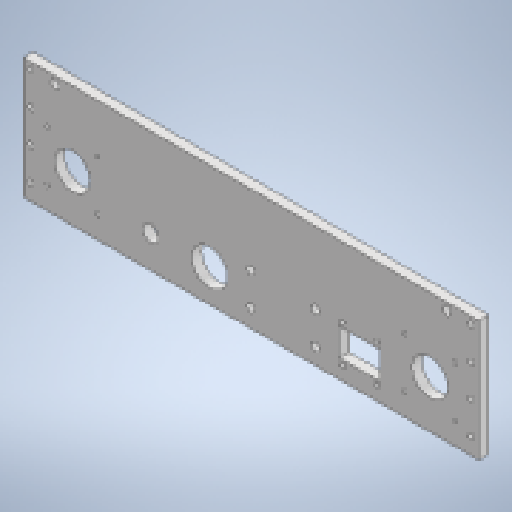
# Autodesk Inventor part: креп_мотора
Saved by Autodesk Inventor 2023.1 (Build 271208000, 208)
## iProperties
Created: 2025-12-22
Part Number: креп_мотора
Material: Типовые
Document SubType Name: Modeling
Designer: DELL
Density: 1 g/cm^3
Appearance: По умолчанию
Author: DELL
Autodesk Inventor part; units mm, degrees
ref_plane "YZ Plane" through (0, 0, 0) normal (1, 0, 0) x (0, 1, 0)
ref_plane "XZ Plane" through (0, 0, 0) normal (0, 1, 0) x (-1, 0, 0)
ref_plane "XY Plane" through (0, 0, 0) normal (0, 0, 1) x (1, 0, 0)
sketch "Эскиз1" plane through (0, 0, 0) normal (0, 0, 1) x (1, 0, 0)
  line L0 (-26.0621, -17.2379) -> (-22.2379, -21.0621) projected
  arc A0 (-22.2379, -21.0621) -> (-22.0257, -21.15) centre (-22.0257, -20.85) ccw projected
  line L1 (-22.0257, -21.15) -> (12.0257, -21.15) projected
  arc A1 (12.0257, -21.15) -> (12.2379, -21.0621) centre (12.0257, -20.85) ccw projected
  line L2 (12.2379, -21.0621) -> (16.0621, -17.2379) projected
  arc A2 (16.0621, -17.2379) -> (16.15, -17.0257) centre (15.85, -17.0257) ccw projected
  line L3 (16.15, -17.0257) -> (16.15, 17.0257) projected
  arc A3 (16.15, 17.0257) -> (16.0621, 17.2379) centre (15.85, 17.0257) ccw projected
  line L4 (16.0621, 17.2379) -> (12.2379, 21.0621) projected
  arc A4 (12.2379, 21.0621) -> (12.0257, 21.15) centre (12.0257, 20.85) ccw projected
  line L5 (12.0257, 21.15) -> (-22.0257, 21.15) projected
  arc A5 (-22.0257, 21.15) -> (-22.2379, 21.0621) centre (-22.0257, 20.85) ccw projected
  line L6 (-22.2379, 21.0621) -> (-26.0621, 17.2379) projected
  arc A6 (-26.0621, 17.2379) -> (-26.15, 17.0257) centre (-25.85, 17.0257) ccw projected
  line L7 (-26.15, 17.0257) -> (-26.15, -17.0257) projected
  arc A7 (-26.15, -17.0257) -> (-26.0621, -17.2379) centre (-25.85, -17.0257) ccw projected
  circle A8 centre (-5, 0) radius 11 projected
  circle A9 centre (-20.5, 15.5) radius 1.25 projected
  circle A10 centre (10.5, 15.5) radius 1.25 projected
  circle A11 centre (10.5, -15.5) radius 1.25 projected
  circle A12 centre (-20.5, -15.5) radius 1.25 projected
  circle A13 centre (20.65, -19.15) radius 1.75 projected
  circle A14 centre (20.65, 0.85) radius 1.75 projected
  circle A15 centre (20.65, 20.85) radius 1.75 projected
  circle A16 centre (20.65, 40.85) radius 1.75 projected
  line L8 (-246.5621, -17.2379) -> (-242.7379, -21.0621) projected
  arc A17 (-242.7379, -21.0621) -> (-242.5257, -21.15) centre (-242.5257, -20.85) ccw projected
  line L9 (-242.5257, -21.15) -> (-208.4743, -21.15) projected
  arc A18 (-208.4743, -21.15) -> (-208.2621, -21.0621) centre (-208.4743, -20.85) ccw projected
  line L10 (-208.2621, -21.0621) -> (-204.4379, -17.2379) projected
  arc A19 (-204.4379, -17.2379) -> (-204.35, -17.0257) centre (-204.65, -17.0257) ccw projected
  line L11 (-204.35, -17.0257) -> (-204.35, 17.0257) projected
  arc A20 (-204.35, 17.0257) -> (-204.4379, 17.2379) centre (-204.65, 17.0257) ccw projected
  line L12 (-204.4379, 17.2379) -> (-208.2621, 21.0621) projected
  arc A21 (-208.2621, 21.0621) -> (-208.4743, 21.15) centre (-208.4743, 20.85) ccw projected
  line L13 (-208.4743, 21.15) -> (-242.5257, 21.15) projected
  arc A22 (-242.5257, 21.15) -> (-242.7379, 21.0621) centre (-242.5257, 20.85) ccw projected
  line L14 (-242.7379, 21.0621) -> (-246.5621, 17.2379) projected
  arc A23 (-246.5621, 17.2379) -> (-246.65, 17.0257) centre (-246.35, 17.0257) ccw projected
  line L15 (-246.65, 17.0257) -> (-246.65, -17.0257) projected
  arc A24 (-246.65, -17.0257) -> (-246.5621, -17.2379) centre (-246.35, -17.0257) ccw projected
  circle A25 centre (-225.5, 0) radius 11 projected
  circle A26 centre (-241, 15.5) radius 1.25 projected
  circle A27 centre (-210, 15.5) radius 1.25 projected
  circle A28 centre (-210, -15.5) radius 1.25 projected
  circle A29 centre (-241, -15.5) radius 1.25 projected
  circle A30 centre (-251.15, -19.15) radius 1.75 projected
  circle A31 centre (-251.15, 0.85) radius 1.75 projected
  circle A32 centre (-251.15, 20.85) radius 1.75 projected
  circle A33 centre (-251.15, 40.85) radius 1.75 projected
  line L16 (-255.45, -29.15) -> (-246.85, -29.15) projected
  line L17 (-255.65, -29.15) -> (-255.65, 270.85) projected
  line L18 (25.15, 270.85) -> (25.15, -29.15) projected
  line L19 (25.15, -29.15) -> (-255.65, -29.15)
  line L20 (-255.65, -29.15) -> (-255.65, 45.35)
  line L21 (-255.65, 45.35) -> (25.15, 45.35)
  line L22 (25.15, 45.35) -> (25.15, -29.15)
  point P0 (25.15, 45.35)
  dimension "d15" = 4.5
  constraints: 8 end point, 2 parallel, 1 horizontal, 1 perpendicular, 1 point on line
  measures "d15" distance from line of L21 A33.centre
extrude "Выдавливание1" add sketch "Эскиз1" along normal blind 6 contours A7 L7 A6 L6 A5 L5 A4 L4 A3 L3 A2 L2 A1 L1 A0 L0 | A24 L15 A23 L14 A22 L13 A21 L12 A20 L11 A19 L10 A18 L9 A17 L8 | L19 L17 L21 L18 L16
sketch "Эскиз2" plane through (0, 0, 6) normal (0, 0, 1) x (1, 0, 0)
  circle A0 centre (20.65, 40.85) radius 1.75 projected
  circle A1 centre (5.65, 40.85) radius 2.6
  circle A2 centre (-236.15, 40.85) radius 2.6
  circle A3 centre (-251.15, 40.85) radius 1.75 projected
  point P0 (0, 0)
  dimension "d16" = 5.2
  dimension "d17" = 15
  dimension "d18" = 5.2
  dimension "d19" = 15
  constraints: 2 centre point
  measures "d16" diameter of A1
  measures "d17" distance of A1.centre A0.centre
  measures "d18" diameter of A2
  measures "d19" distance of A3.centre A2.centre
extrude "Выдавливание2" cut sketch "Эскиз2" against normal blind 6
sketch "Эскиз3" plane through (0, 0, 0) normal (0, 0, -1) x (-1, 0, 0)
  circle A0 centre (115.25, -18.05) radius 2.55
  circle A1 centre (115.25, 1.95) radius 2.55
  line L0 (255.65, 45.35) -> (255.65, -29.15) projected
  point P0 (0, 0)
  dimension "d25" = 5.1
  dimension "d26" = 140.4
  dimension "d27" = 140.4
  constraints: 2 centre point
  measures "d25" diameter of A0
  measures "d26" distance from line of L0 A0.centre
  measures "d27" distance from line of L0 A1.centre
extrude "Выдавливание3" cut sketch "Эскиз3" against normal blind 10
sketch "Эскиз4" plane through (0, 0, 6) normal (0, 0, 1) x (1, 0, 0)
  circle A0 centre (-177.15, -2.65) radius 5 construction
  line L0 (-177.15, -2.65) -> (-177.15, -29.15) construction
  line L1 (-255.65, -29.15) -> (25.15, -29.15) construction
  circle A1 centre (-177.15, -9.15) radius 5
  point P0 (0, 0)
  dimension "d30" = 10
  dimension "d31" = 20
  constraints: 2 centre point, 2 end point, 2 point on line, 1 vertical
  measures "d30" diameter of A1
  measures "d31" distance from line of L1 A1.centre
extrude "Выдавливание4" cut sketch "Эскиз4" against normal blind 10
sketch "Эскиз5" plane through (0, 0, 6) normal (0, 0, 1) x (1, 0, 0)
  circle A0 centre (-20.5, 15.5) radius 1.25 construction
  circle A1 centre (-20.5, -15.5) radius 1.25 construction
  circle A2 centre (-20.5, -15.5) radius 1.25 projected
  circle A3 centre (-20.5, 15.5) radius 1.25 projected
  line L0 (-20.5, -15.5) -> (-20.5, 15.5) construction
  line L1 (-60.8, -17.65) -> (-35.5, -17.65)
  line L2 (-35.5, -17.65) -> (-35.5, -0.65)
  line L3 (-35.5, -0.65) -> (-60.8, -0.65)
  line L4 (-60.8, -0.65) -> (-60.8, -17.65)
  line L5 (-60.8, -17.65) -> (-35.5, -0.65) construction
  line L6 (-35.5, -17.65) -> (-60.8, -0.65) construction
  circle A4 centre (-58.8, -20.9) radius 1.35
  line L7 (-48.15, -9.15) -> (-48.15, -2.4897)
  line L8 (-48.15, -9.15) -> (-50.139, -9.15)
  circle A5 centre (-37.5, -20.9) radius 1.35
  circle A6 centre (-58.8, 2.6) radius 1.35
  circle A7 centre (-37.5, 2.6) radius 1.35
  line L9 (-255.65, -29.15) -> (25.15, -29.15) projected
  point P0 (0, 0)
  dimension "d33" = 17
  dimension "d39" = 2.7
  dimension "d40" = 3.25
  dimension "d41" = 2
  dimension "d45" = 25.3
  dimension "d46" = 20
  constraints: 18 end point, 4 centre point, 3 symmetric about line, 2 midpoint, 2 parallel, 1 horizontal, 1 perpendicular, 1 vertical, 3 other
  measures "d33" distance of L2.end L1.end
  measures "d39" diameter of A4
  measures "d40" distance from line of L1 A4.centre
  measures "d41" distance from line of L4 A4.centre
  measures "d45" distance between parallel lines of L2 L4
  measures "d46" distance from line of L9 L7.start
extrude "Выдавливание5" cut sketch "Эскиз5" against normal blind 10
sketch "Эскиз6" plane through (0, 0, 6) normal (0, 0, 1) x (1, 0, 0)
  line L0 (-60.8, -17.65) -> (-60.8, -0.65) construction
  line L1 (-60.8, -9.15) -> (-101.8454, -9.15) construction
  circle A0 centre (-75.8, -19.15) radius 2.55
  circle A1 centre (-75.8, 0.85) radius 2.55
  line L2 (-75.8, 0.85) -> (-75.8, -20.3687) construction
  line L3 (-101.8454, -9.15) -> (-167.9603, -9.15) construction
  circle A2 centre (-140.8, -9.15) radius 11
  point P0 (0, 0)
  dimension "d47" = 5.1
  dimension "d48" = 5.1
  dimension "d49" = 10
  dimension "d50" = 10
  dimension "d51" = 15
  dimension "d54" = 22
  dimension "d55" = 65
  constraints: 6 end point, 3 centre point, 2 horizontal, 2 point on line, 1 midpoint, 1 vertical
  measures "d47" diameter of A0
  measures "d48" diameter of A1
  measures "d49" distance from line of A0.centre L1
  measures "d50" distance from line of L2.start L1
  measures "d51" distance between parallel lines of L0 L2
  measures "d54" diameter of A2
  measures "d55" distance from line of L2 A2.centre
extrude "Выдавливание6" cut sketch "Эскиз6" against normal blind 10
